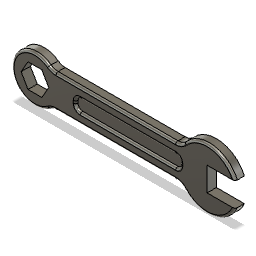
Wrench v5 (Autodesk Fusion 360 design; units mm, degrees)
Autodesk Fusion 360 part; units mm, degrees
sketch "Sketch1" plane through (0, 0, 0) normal (0, 0, 1) x (1, 0, 0)
  line L0 (-37.0266, -5.15) -> (-34.0533, 0)
  line L1 (-34.0533, 0) -> (-37.0266, 5.15)
  line L2 (-37.0266, 5.15) -> (-42.9734, 5.15)
  line L3 (-42.9734, 5.15) -> (-45.9467, 0)
  line L4 (-45.9467, 0) -> (-42.9734, -5.15)
  line L5 (-42.9734, -5.15) -> (-37.0266, -5.15)
  line L6 (46, -5.15) -> (34, -5.15)
  line L7 (34, -5.15) -> (34, 5.15)
  line L8 (34, 5.15) -> (46, 5.15)
  line L9 (46, -5.15) -> (34, 5.15) construction
  line L10 (34, -5.15) -> (46, 5.15) construction
  line L11 (-32.8586, 7) -> (22.9763, 7)
  line L12 (-32.8586, -7) -> (22.9763, -7)
  arc A0 (-32.8586, 7) -> (-32.8586, -7) centre (-40, 0) ccw
  arc A1 (22.9763, -7) -> (46, -5.15) centre (34, 0) ccw
  arc A2 (46, 5.15) -> (22.9763, 7) centre (34, 0) ccw
  point P0 (-40, 0)
  point P1 (40, 0)
  dimension "d1" = 80
  dimension "d2" = 5.15
  dimension "d3" = 20
  dimension "d4" = 12
  dimension "d5" = 10.3
  constraint horizontal L2
  constraint coincident P0 A0.centre
  constraint horizontal L6
  constraint perpendicular L6 L7
  constraint parallel L6 L8
  constraint coincident L9 P1
  constraint coincident L10 P1
  constraint midpoint L7 A1.centre
  constraint coincident L8.end A1
  constraint concentric A1 A2
  measures "d1" distance of P0 P1
  measures "d2" distance of P0 L5
  measures "d3" diameter of A0
  measures "d4" distance of L7.end L8.end
  measures "d5" distance of L6.end L7.end
extrude "Extrude1" add sketch "Sketch1" along normal blind 4
fillet "Fillet1" radius 5 4 edges at (-32.8586, 7, 2) (22.9763, 7, 2) (22.9763, -7, 2) (-32.8586, -7, 2)
sketch "Sketch2" plane through (0, 0, 4) normal (0, 0, 1) x (1, 0, 0)
  line L0 (-37.0266, -5.15) -> (-42.9734, -5.15)
  line L1 (-42.9734, -5.15) -> (-45.9467, 0)
  line L2 (-45.9467, 0) -> (-42.9734, 5.15)
  line L3 (-42.9734, 5.15) -> (-37.0266, 5.15)
  line L4 (-37.0266, 5.15) -> (-34.0533, 0)
  line L5 (-34.0533, 0) -> (-37.0266, -5.15)
  arc A0 (-34, 8) -> (-34, -8) centre (-40, 0) ccw
  arc A1 (-31, -7) -> (-34, -8) centre (-31, -12) ccw
  line L6 (-31, -7) -> (20.5053, -7)
  arc A2 (24.2417, -8.6775) -> (20.5053, -7) centre (20.5053, -12) ccw
  arc A3 (24.2417, -8.6775) -> (46, -5.15) centre (34, 0) ccw
  line L7 (46, -5.15) -> (34, -5.15)
  line L8 (34, -5.15) -> (34, 5.15)
  line L9 (34, 5.15) -> (46, 5.15)
  arc A4 (46, 5.15) -> (24.2417, 8.6775) centre (34, 0) ccw
  arc A5 (20.5053, 7) -> (24.2417, 8.6775) centre (20.5053, 12) ccw
  line L10 (20.5053, 7) -> (-31, 7)
  arc A6 (-34, 8) -> (-31, 7) centre (-31, 12) ccw
  line L11 (20.5, -2.5) -> (-20.5, -2.5)
  line L12 (-22.5, -0.5) -> (-22.5, 0.5)
  line L13 (-20.5, 2.5) -> (20.5, 2.5)
  line L14 (22.5, 0.5) -> (22.5, -0.5)
  line L15 (22.5, -2.5) -> (-22.5, 2.5) construction
  line L16 (-22.5, -2.5) -> (22.5, 2.5) construction
  arc A7 (-20.5, 2.5) -> (-22.5, 0.5) centre (-20.5, 0.5) ccw
  arc A8 (-22.5, -0.5) -> (-20.5, -2.5) centre (-20.5, -0.5) ccw
  arc A9 (22.5, 0.5) -> (20.5, 2.5) centre (20.5, 0.5) ccw
  arc A10 (20.5, -2.5) -> (22.5, -0.5) centre (20.5, -0.5) ccw
  dimension "d12" = 45
  dimension "d13" = 5
  dimension "d14" = 2
  constraint horizontal L11
  constraint perpendicular L11 L12
  constraint parallel L11 L13
  constraint parallel L12 L14
  constraint coincident L15 origin
  constraint coincident L16 origin
  constraint coincident L15.end L13
  constraint coincident L15.end L12
  constraint tangent L13 A7
  constraint tangent L12 A7
  constraint coincident L16.start L11
  constraint coincident L16.start L12
  constraint tangent L11 A8
  constraint tangent L12 A8
  constraint equal A7 A8
  constraint coincident L16.end L13
  constraint coincident L16.end L14
  constraint tangent L13 A9
  constraint tangent L14 A9
  constraint equal A7 A9
  constraint coincident L15.start L11
  constraint coincident L15.start L14
  constraint tangent L11 A10
  constraint tangent L14 A10
  constraint equal A7 A10
  measures "d12" distance of L15.end L16.end
  measures "d13" distance of L16.start L15.end
  measures "d14" radius of A7
extrude "Extrude2" cut sketch "Sketch2" against normal blind 1 contours L11 L12 L13 L14 A7 A8 A9 A10
fillet "Fillet2" radius 1 17 edges at (22.5, 0, 4) (21.9142, -1.9142, 4) (0, -2.5, 4) (-21.9142, -1.9142, 4) (-22.5, 0, 4) (-21.9142, 1.9142, 4) (0, 2.5, 4) (21.9142, 1.9142, 4) (36.0897, 12.8901, 4) (22.5531, 7.4386, 4) (-5.2473, 7, 4) (-32.5811, 7.2566, 4) (-50, 0, 4) (-32.5811, -7.2566, 4) (-5.2473, -7, 4) (22.5531, -7.4386, 4) (36.0897, -12.8901, 4)
